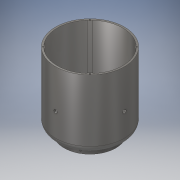
# Autodesk Inventor part: Avi Bay Steel
Saved by Autodesk Inventor 2017 (Build 210142000, 142)
## iProperties
Created: 2016-11-08
Part Number: Avi Bay Steel
Material: Steel, Carbon
Document SubType Name: Modeling
Designer: mnweir
Density: 7.85 g/cm^3
Appearance: Semi-Polished
Author: mnweir
Autodesk Inventor part; units mm, degrees
ref_plane "XZ Plane" through (0, 0, 0) normal (0, 1, 0) x (-1, 0, 0)
sketch "Sketch1" plane through (0, 0, 0) normal (0, 0, 1) x (1, 0, 0)
  line L0 (0, 151.2794) -> (0, -132.7897) construction
  line L1 (-127, 143.1042) -> (-127, -85.4958)
  line L2 (-127, -85.4958) -> (-101.6, -85.4958) construction
  line L3 (-101.6, -85.4958) -> (-101.6, -110.8958) construction
  arc A0 (-127, -85.4958) -> (-101.6, -110.8958) centre (-101.6, -85.4958) ccw
  line L4 (-101.6, -110.8958) -> (0, -110.8958)
  line L5 (-95.25, -132.7897) -> (-88.9, -132.7897)
  line L6 (-88.9, -132.7897) -> (-88.9, -110.8958)
  line L7 (-127, 143.1042) -> (-114.3, 143.1042)
  line L8 (-114.3, 143.1042) -> (-114.3, -85.4958)
  arc A1 (-114.3, -85.4958) -> (-101.6, -98.1958) centre (-101.6, -85.4958) ccw
  line L9 (-101.6, -98.1958) -> (0, -98.1958)
  line L10 (0, -98.1958) -> (0, -110.8958)
  line L11 (-95.25, -132.7897) -> (-95.25, -110.8958)
  point P0 (0, 0)
  dimension "d0" = 228.6
  dimension "d1" = 127
  dimension "d2" = 25.4
  dimension "d3" = 110.8958
  dimension "d4" = 262.1752
  dimension "d5" = 21.8939
  dimension "d6" = 88.9
  dimension "d8" = 21.8939
  dimension "d16" = 12.7
  dimension "d22" = 95.25
  constraints: 24 end point, 6 perpendicular, 4 point on circle, 4 point on line, 2 centre point, 2 coincident, 2 horizontal, 2 vertical, 1 collinear, 1 midpoint, 1 tangent
  measures "d0" distance of L1.start L1.end
  measures "d1" distance between parallel lines of L0 L1
  measures "d2" distance of L1.end L2.end
  measures "d3" distance from line of point (0, 0) L4
  measures "d4" distance from line of L0.start L4
  measures "d5" distance from line of L0.end L4
  measures "d6" distance between parallel lines of L6 L0
  measures "d8" distance between parallel lines of L5 L4
  measures "d16" distance of L1.start L7.end
  measures "d22" distance between parallel lines of L11 L0
revolve "Revolution1" add sketch "Sketch1" angle 360 about axis through (0, 151.2794, 0) along (0, -1, 0)
fillet "Fillet1" radius 3.175 1 edges at (95.25, -110.8958, 0)
ref_plane "Work Plane1" through (-95.25, -121.8427, 0) normal (1, 0, 0) x (0, 1, 0)
sketch "Sketch2" plane through (-95.25, -121.8427, 0) normal (1, 0, 0) x (0, 1, 0)
  line L0 (121.8427, 0) -> (-1.3473, 0) construction
  dimension "d24" = 123.19
  constraints: 2 end point, 1 horizontal
  measures "d24" distance of L0.start L0.end
hole "Hole1" at (-95.25, -123.19, 0) direction (1, 0, 0) diameter 4.9784 depth 19.05 tip angle 118 thread size "1/4-20 UNC" class "2B" standard "ANSI Unified Screw Threads"
pattern_circular "Circular Pattern1" count 6 over 360 about axis through (0, -10, 0) along (0, 1, 0) of "Hole1"
ref_plane "Work Plane2" through (0, 28.8042, -127) normal (0, 0, 1) x (1, 0, 0)
sketch "Sketch3" plane through (0, 28.8042, -127) normal (0, 0, 1) x (1, 0, 0)
  point P0 (0, -28.8042)
  point P1 (0, -28.8042)
  constraints: 1 coincident
hole "Hole2" at (0, 0, -127) direction (0, 0, 1) diameter 12.7 depth 19.05 tip angle 118
pattern_circular "Circular Pattern2" count 4 over 360 about axis through (0, -10, 0) along (0, 1, 0) of "Hole2"
sketch "Sketch4" plane through (0, -98.1958, 0) normal (0, 1, 0) x (1, 0, 0)
  circle A0 centre (0, 0) radius 9.525
  dimension "d45" = 19.05
  constraints: 1 centre point, 1 coincident
  measures "d45" diameter of A0
extrude "Extrusion1" cut sketch "Sketch4" against normal blind 42.8625
sketch "Sketch5" plane through (0, 143.1042, 0) normal (0, 1, 0) x (1, 0, 0)
  circle A0 centre (0, 0) radius 120.65
  dimension "d48" = 241.3
  constraints: 1 centre point, 1 coincident
  measures "d48" diameter of A0
extrude "Extrusion2" cut sketch "Sketch5" against normal blind 228.6
sketch "Sketch6" plane through (0, 143.1042, 0) normal (0, 1, 0) x (1, 0, 0)
  circle A0 centre (0, 0) radius 9.525 projected
  circle A1 centre (0, 0) radius 120.65 projected
  line L0 (0, 0) -> (0, -181.3672) construction
  line L1 (0, 0) -> (-85.3124, -85.3124)
  line L2 (-82.3442, -92.5841) -> (-78.0408, -88.2806)
  line L3 (-78.0408, -88.2806) -> (-88.2806, -78.0408)
  line L4 (-88.2806, -78.0408) -> (-92.5841, -82.3442)
  line L5 (-92.5841, -82.3442) -> (-82.3442, -92.5841)
  line L6 (-82.3442, -92.5841) -> (-88.2806, -78.0408) construction
  line L7 (-78.0408, -88.2806) -> (-92.5841, -82.3442) construction
  dimension "d53" = 45
  dimension "d54" = 4.3035
  constraints: 16 end point, 2 midpoint, 2 parallel, 1 perpendicular, 1 vertical, 2 other
  measures "d53" angle of L0 L1
  measures "d54" horizontal distance of L2.start L2.end
extrude "Extrusion3" add sketch "Sketch6" against normal blind 228.6 contours L3 L2 A1 L1 | L1 A1 L4 L3 | A1 L2 L5 L4
pattern_circular "Circular Pattern3" count 4 over 360 about axis through (0, -10, 0) along (0, 1, 0) of "Extrusion3"
sketch "Sketch11" plane through (0, 143.1042, 0) normal (0, 1, 0) x (1, 0, 0)
  line L0 (0, 0) -> (86.3822, -86.3822) construction
  line L1 (78.0408, -88.2806) -> (88.2806, -78.0408) projected
  constraints: 2 end point, 1 perpendicular
hole "Hole7" at (86.3822, 143.1042, 86.3822) direction (0, -1, 0) diameter 4.9784 depth 19.05 tip angle 118 thread size "1/4-20 UNC" class "2B" standard "ANSI Unified Screw Threads"
pattern_circular "Circular Pattern4" count 4 over 360 about axis through (0, -10, 0) along (0, 1, 0) of "Hole7"
body "Solid1"
